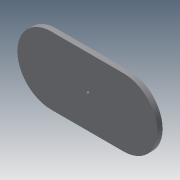
# Autodesk Inventor part: deska_pod_rameno
Saved by Autodesk Inventor 2013 (Build 170138000, 138)
## iProperties
Created: 2013-06-08
Part Number: deska_pod_rameno
Material: Generic
Document SubType Name: Modeling
Designer: idle-rug
Density: 1 g/cm^3
Author: idle-rug
Autodesk Inventor part; units mm, degrees
ref_plane "YZ Plane" through (0, 0, 0) normal (1, 0, 0) x (0, 1, 0)
ref_plane "XZ Plane" through (0, 0, 0) normal (0, 1, 0) x (-1, 0, 0)
ref_plane "XY Plane" through (0, 0, 0) normal (0, 0, 1) x (1, 0, 0)
sketch "Sketch1" plane through (0, 0, 0) normal (0, 1, 0) x (-1, 0, 0)
  line L0 (70, 65.5) -> (-70, 65.5)
  line L1 (-70, 65.5) -> (-70, -65.5)
  line L2 (-70, -65.5) -> (70, -65.5)
  line L3 (70, -65.5) -> (70, 65.5)
  line L4 (70, 65.5) -> (-70, -65.5) construction
  line L5 (-70, 65.5) -> (70, -65.5) construction
  circle A0 centre (0, 0) radius 7.5
  dimension "d0" = 140
  dimension "d1" = 131
  dimension "d2" = 15
  constraints: 12 end point, 2 midpoint, 2 parallel, 1 centre point, 1 coincident, 1 horizontal, 1 perpendicular
  measures "d0" distance of L2.end L1.end
  measures "d1" distance of L1.end L0.end
  measures "d2" diameter of A0
extrude "Extrusion1" add sketch "Sketch1" along normal blind 10
sketch "Sketch2" plane through (0, 10, 0) normal (0, 1, 0) x (1, 0, 0)
  circle A0 centre (0, 0) radius 7.5 projected
  circle A1 centre (0, 0) radius 3
  dimension "d5" = 6
  constraints: 1 centre point, 1 coincident
  measures "d5" diameter of A1
extrude "Extrusion2" add sketch "Sketch2" against normal blind 10
sketch "Sketch3" plane through (0, 10, 0) normal (0, 1, 0) x (1, 0, 0)
  line L0 (70, -65.5) -> (70, 65.5) projected
  line L1 (-70, 65.5) -> (-70, -65.5) projected
  arc A0 (70, -65.5) -> (70, 65.5) centre (-5.5629, 0) ccw
  arc A1 (-70, 65.5) -> (-70, -65.5) centre (5.5629, 0) ccw
  dimension "d10" = 100
  dimension "d11" = 100
  constraints: 4 point on circle, 2 centre point
  measures "d10" radius of A0
  measures "d11" radius of A1
extrude "Extrusion3" add sketch "Sketch3" against normal blind 10
body "Solid1"
